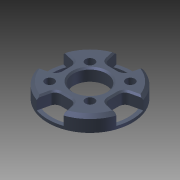
# Autodesk Inventor part: base
Saved by Autodesk Inventor 2012 (Build 160160000, 160)
## iProperties
Created: 2014-07-09
Part Number: base
Material: Default
Document SubType Name: Modeling
Designer: Anon
Density: 1 g/cm^3
Author: Anon
Autodesk Inventor part; units mm, degrees
ref_plane "YZ Plane" through (0, 0, 0) normal (1, 0, 0) x (0, 1, 0)
ref_plane "XZ Plane" through (0, 0, 0) normal (0, 1, 0) x (-1, 0, 0)
sketch "Sketch1" plane through (0, 0, 0) normal (0, 0, 1) x (1, 0, 0)
  circle A0 centre (0, 0) radius 14
  dimension "d0" = 28
  constraints: 1 centre point, 1 coincident
  measures "d0" diameter of A0
extrude "Extrusion1" add sketch "Sketch1" along normal blind 5
chamfer "Chamfer1" distance 1 angle 45 1 edges at (-14, 0, 5)
ref_plane "Work Plane1" through (0, 0, 1) normal (0, 0, 1) x (1, 0, 0)
sketch "Sketch2" plane through (0, 0, 1) normal (0, 0, 1) x (1, 0, 0)
  line L0 (8, 3.25) -> (8, -3.25)
  line L1 (8, 3.25) -> (14.5, 4.75)
  line L2 (14.5, 4.75) -> (14.5, -4.75)
  line L3 (14.5, -4.75) -> (8, -3.25)
  point P0 (0, 0)
  dimension "d7" = 8
  dimension "d8" = 6.5
  dimension "d9" = 3.25
  dimension "d10" = 9.5
  dimension "d11" = 4.75
  dimension "d12" = 6.5
  constraints: 8 end point, 1 parallel, 1 vertical
  measures "d7" distance from line of point (0, 0) L0
  measures "d8" distance of L0.end L0.start
  measures "d9" vertical distance of point (0, 0) L0.end
  measures "d10" distance of L2.end L1.end
  measures "d11" vertical distance of point (0, 0) L1.end
  measures "d12" distance between parallel lines of L2 L0
extrude "Extrusion2" cut sketch "Sketch2" along normal blind 5
fillet "Fillet1" radius 2 2 edges at (8, 3.25, 3) (8, -3.25, 3)
chamfer "Chamfer2" distance 0.5 angle 45 5 edges at (10.9197, 3.9238, 5) (8.4348, 2.9041, 5) (8, 0, 5) (8.4348, -2.9041, 5) (10.9197, -3.9238, 5)
pattern_circular "Circular Pattern1" count 4 over 360 about axis through (0, 0, -10) along (0, 0, 1) of "Extrusion2", "Fillet1", "Chamfer2"
sketch "Sketch3" plane through (0, 0, 0) normal (0, 0, -1) x (-1, 0, 0)
  circle A0 centre (0, 0) radius 14 projected
  circle A1 centre (0, 0) radius 12.7
  dimension "d22" = 1.3
  constraints: 1 centre point, 1 coincident
  measures "d22" radial gap between concentric circles of A0 A1
extrude "Extrusion3" cut sketch "Sketch3" against normal blind 1 contours A1
sketch "Sketch4" plane through (0, 0, 5) normal (0, 0, 1) x (1, 0, 0)
  arc A0 (-12.1156, -4.7129) -> (-4.7129, -12.1156) centre (0, 0) ccw projected
  constraints: 1 coincident
hole "Hole1" at (0, 0, 5) direction (0, 0, -1) diameter 11 end through all
chamfer "Chamfer3" distance 0.5 angle 45 1 edges at (0, 5.5, 5)
sketch "Sketch5" plane through (0, 0, 5) normal (0, 0, 1) x (1, 0, 0)
  line L0 (1.659, -7.5) -> (-1.659, -7.5) projected
  circle A0 centre (0, 0) radius 6 projected
  line L1 (0, 0) -> (-5.6569, 5.6569)
  line L2 (0, 0) -> (-17.4716, 0) construction
  line L3 (0, 0) -> (5.6569, -5.6569) construction
  line L4 (0, 0) -> (6.7175, 6.7175) construction
  line L5 (0, 0) -> (-6.7175, -6.7175) construction
  dimension "d35" = 8
  dimension "d36" = 45
  dimension "d37" = 8
  dimension "d38" = 9.5
  dimension "d39" = 9.5
  constraints: 10 end point, 4 coincident, 2 collinear, 1 parallel, 1 perpendicular
  measures "d35" distance of L1.start L1.end
  measures "d36" angle of L2 L1
  measures "d37" distance of L1.start L3.end
  measures "d38" distance of L1.start L4.end
  measures "d39" distance of L1.start L5.end
hole "Hole2" at (-5.6569, 5.6569, 5) at (5.6569, -5.6569, 5) at (-6.7175, -6.7175, 5) at (6.7175, 6.7175, 5) direction (0, 0, -1) diameter 3 end through all
body "Solid1"
